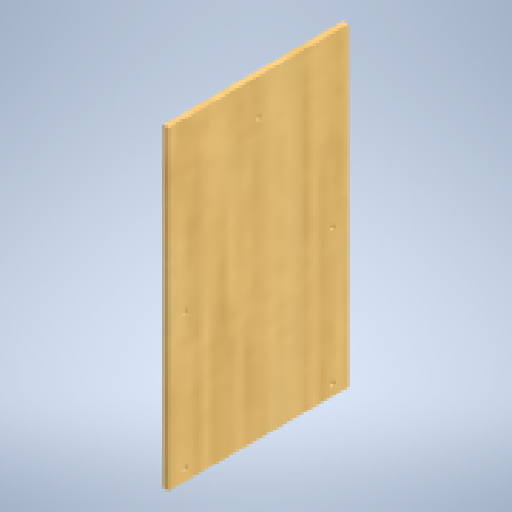
# Autodesk Inventor part: Panel4
Saved by Autodesk Inventor 2023 (Build 270158000, 158)
## iProperties
Created: 2022-12-03
Part Number: Panel4
Material: Genérico
Document SubType Name: Modeling
Designer: sergi
Density: 1 g/cm^3
Appearance: Valor por defecto
Author: sergi
Autodesk Inventor part; units mm, degrees
ref_plane "YZ Plane" through (0, 0, 0) normal (1, 0, 0) x (0, 1, 0)
ref_plane "XZ Plane" through (0, 0, 0) normal (0, 1, 0) x (-1, 0, 0)
ref_plane "XY Plane" through (0, 0, 0) normal (0, 0, 1) x (1, 0, 0)
sketch "Boceto1" plane through (0, 0, 0) normal (0, 1, 0) x (-1, 0, 0)
  line L0 (-1.5, -51.5) -> (1.5, -51.5)
  line L1 (1.5, -51.5) -> (1.5, 51.5)
  line L2 (1.5, 51.5) -> (-1.5, 51.5)
  line L3 (-1.5, 51.5) -> (-1.5, -51.5)
  line L4 (-1.5, -51.5) -> (1.5, 51.5) construction
  line L5 (1.5, -51.5) -> (-1.5, 51.5) construction
  point P0 (0, 0)
  dimension "d0" = 3
  dimension "d1" = 103
  constraints: 12 end point, 2 midpoint, 2 parallel, 1 horizontal, 1 perpendicular
  measures "d0" distance of L2.end L1.end
  measures "d1" distance of L1.end L0.end
extrude "Extrusión1" add sketch "Boceto1" along normal blind 180
sketch "Boceto2" plane through (-1.5, 0, -51.5) normal (-1, 0, 0) x (0, 0, 1)
  circle A0 centre (9.5, 6.5) radius 1.25 projected
  circle A1 centre (93.5, 6.5) radius 1.25 projected
  line L0 (103, 0) -> (0, 0) projected
  line L1 (0, 0) -> (0, 180) projected
  line L2 (103, 180) -> (0, 180) projected
  line L3 (103, 0) -> (103, 180) projected
  line L4 (0, 0) -> (103, 0) projected
  line L5 (103, 0) -> (103, 180) projected
  line L6 (0, 180) -> (103, 180) projected
  line L7 (0, 0) -> (0, 180) projected
  line L8 (0, 0) -> (0, 180) projected
  circle A2 centre (51.5, 159.25) radius 1.25 projected
  circle A3 centre (93.5, 84) radius 1.5 projected
  circle A4 centre (9.5, 84) radius 1.5 projected
  point P0 (51.5, 0)
hole "Agujero1" at (-1.5, 84, -42) at (-1.5, 6.5, -42) at (-1.5, 6.5, 42) at (-1.5, 84, 42) at (-1.5, 159.25, 0) direction (1, 0, 0) diameter 3 depth 5 tip angle 118
